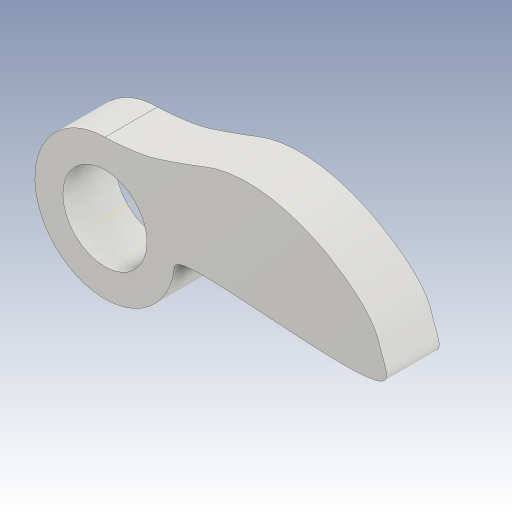
# Autodesk Inventor part: Kurvenscheibe
Saved by Autodesk Inventor 2023.3 (Build 273359000, 359)
## iProperties
CustomPartVersion: 1
Created: 2024-06-19
Part Number: Kurvenscheibe
Material: Stainless Steel, Austenitic
Document SubType Name: Modeling
Designer: nicob
Manufacturer: Standard
Standards Organization: Custom
Mass: 2.33722 g
Surface Area: 3.89592 cm^2
Volume: 0.292153 cm^3
Density: 8 g/cm^3
Appearance: Steel
Author: nicob
Autodesk Inventor part; units mm, degrees
ref_plane "YZ Plane" through (0, 0, 0) normal (1, 0, 0) x (0, 1, 0)
ref_plane "XZ Plane" through (0, 0, 0) normal (0, 1, 0) x (-1, 0, 0)
ref_plane "XY Plane" through (0, 0, 0) normal (0, 0, 1) x (1, 0, 0)
sketch "Hauptskizze" plane through (0, 0, 0) normal (0, 0, 1) x (1, 0, 0)
  spline S0 degree 5 poles (0, 4) (0.2649, 4.0101) (0.8873, 4.0398) (2.515, 4.192) (3.2797, 4.5549) (4.8019, 5.0019) (6.0713, 5.5708) (6.9056, 5.7677) (8.0517, 5.8923) (9.1641, 5.8106) (10.3651, 5.5838) (11.6027, 5.1407) (12.7547, 4.5865) (14.071, 3.7053) (14.9564, 2.9343) (15.8723, 1.7782) (15.557, 0.6448) (18.2636, -1.3619) (2.9211, 0.6129) (4.1603, -0.3906) (3.8647, -1.0183) (3.7046, -1.5675) (3.4711, -2.005) (3.246, -2.3578) (2.9803, -2.6838) (2.6841, -2.9808) (2.3575, -3.2449) (2.0055, -3.4736) (1.6314, -3.6642) (1.2395, -3.8147) (0.8339, -3.9233) (0.4193, -3.989) (0, -4.011) (-0.4193, -3.989) (-0.8339, -3.9233) (-1.2395, -3.8147) (-1.6314, -3.6642) (-2.0055, -3.4736) (-2.3576, -3.245) (-2.6839, -2.9807) (-2.9807, -2.6839) (-3.245, -2.3576) (-3.4736, -2.0055) (-3.6642, -1.6314) (-3.8147, -1.2395) (-3.9233, -0.8339) (-3.989, -0.4193) (-4.011, 0) (-3.989, 0.4193) (-3.9233, 0.8339) (-3.8147, 1.2395) (-3.6642, 1.6314) (-3.4737, 2.0055) (-3.2449, 2.3576) (-2.9809, 2.6838) (-2.6834, 2.9808) (-2.3587, 3.2448) (-2.0029, 3.474) (-1.6374, 3.6633) (-1.242, 3.8107) (-0.8802, 3.9148) (-0.4716, 3.9809) (-0.2994, 3.99) (-0.1296, 3.9951) (0, 4) knots 0 0 0 0 0 0 0.032527 0.053166 0.077662 0.100621 0.122564 0.143987 0.165445 0.187942 0.211435 0.235096 0.258425 0.281208 0.30325 0.334435 0.363802 0.391646 0.417983 0.442818 0.456084 0.46935 0.482616 0.495883 0.509149 0.522415 0.535681 0.548948 0.562214 0.57548 0.588746 0.602013 0.615279 0.628545 0.641811 0.655078 0.668344 0.68161 0.694876 0.708143 0.721409 0.734675 0.747941 0.761208 0.774474 0.78774 0.801006 0.814273 0.827539 0.840805 0.854071 0.867338 0.880604 0.89387 0.907136 0.920403 0.933669 0.946935 0.960201 0.973468 0.984081 1 1 1 1 1 1
  point P0 (3.5001, 4.5934)
  point P1 (4.9198, 5.0905)
  point P2 (6.1373, 5.5405)
  point P3 (6.9964, 5.7503)
  point P4 (7.9845, 5.842)
  point P5 (9.0837, 5.7865)
  point P6 (10.2709, 5.5585)
  point P7 (11.519, 5.1367)
  point P8 (12.7972, 4.5047)
  point P9 (14.0723, 3.6509)
  point P10 (14.9501, 2.8498)
  point P11 (15.5253, 1.9865)
  point P12 (15.88, 1.0198)
  point P13 (16, 0)
  point P14 (3.9781, -0.4181)
  point P15 (3.9126, -0.8316)
  point P16 (3.8042, -1.2361)
  point P17 (3.6542, -1.6269)
  point P18 (3.4641, -2)
  point P19 (3.2361, -2.3511)
  point P20 (2.9726, -2.6765)
  point P21 (2.6765, -2.9726)
  point P22 (2.3511, -3.2361)
  point P23 (2, -3.4641)
  point P24 (1.6269, -3.6542)
  point P25 (1.2361, -3.8042)
  point P26 (0.8316, -3.9126)
  point P27 (0.4181, -3.9781)
  point P28 (0, -4)
  point P29 (-0.4181, -3.9781)
  point P30 (-0.8316, -3.9126)
  point P31 (-1.2361, -3.8042)
  point P32 (-1.6269, -3.6542)
  point P33 (-2, -3.4641)
  point P34 (-2.3511, -3.2361)
  point P35 (-2.6765, -2.9726)
  point P36 (-2.9726, -2.6765)
  point P37 (-3.2361, -2.3511)
  point P38 (-3.4641, -2)
  point P39 (-3.6542, -1.6269)
  point P40 (-3.8042, -1.2361)
  point P41 (-3.9126, -0.8316)
  point P42 (-3.9781, -0.4181)
  point P43 (-4, 0)
  point P44 (-3.9781, 0.4181)
  point P45 (-3.9126, 0.8316)
  point P46 (-3.8042, 1.2361)
  point P47 (-3.6542, 1.6269)
  point P48 (-3.4641, 2)
  point P49 (-3.2361, 2.3511)
  point P50 (-2.9726, 2.6765)
  point P51 (-2.6765, 2.9726)
  point P52 (-2.3511, 3.2361)
  point P53 (-2, 3.4641)
  point P54 (-1.6269, 3.6542)
  point P55 (-1.2361, 3.8042)
  point P56 (-0.8316, 3.9126)
  point P57 (-0.4181, 3.9781)
  constraints: 60 other
extrude "Nocken" add sketch "Hauptskizze" along normal blind 3
sketch "Skizze2" plane through (0, 0, 3) normal (0, 0, 1) x (1, 0, 0)
  point P0 (0, 0)
hole "Bohrung1" at (0, 0, 3) direction (0, 0, -1) diameter 4.8 depth 8.8
body "Solid1"
